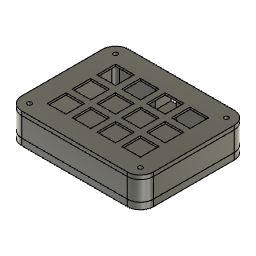
Final_Project (Autodesk Fusion 360 design; units mm, degrees)
Autodesk Fusion 360 part; units mm, degrees
note: some values were not read from the file. Chosen so that the rebuilt part matches the saved one: which bodies a step acts on.
sketch "Sketch1" plane through (0, 0, 0) normal (0, 0, 1) x (1, 0, 0)
  line L0 (-50.425, 81.85) -> (50.425, 81.85)
  line L1 (50.425, 81.85) -> (50.425, 0)
  line L2 (50.425, 0) -> (-50.425, 0)
  line L3 (-50.425, 0) -> (-50.425, 81.85)
  line L4 (-35.425, 28.85) -> (-21.575, 28.85)
  line L5 (-21.575, 28.85) -> (-21.575, 15)
  line L6 (-21.575, 15) -> (-35.425, 15)
  line L7 (-35.425, 15) -> (-35.425, 28.85)
  line L8 (-16.425, 28.85) -> (-2.575, 28.85)
  line L9 (-2.575, 28.85) -> (-2.575, 15)
  line L10 (-2.575, 15) -> (-16.425, 15)
  line L11 (-16.425, 15) -> (-16.425, 28.85)
  line L12 (2.575, 28.85) -> (16.425, 28.85)
  line L13 (16.425, 28.85) -> (16.425, 15)
  line L14 (16.425, 15) -> (2.575, 15)
  line L15 (2.575, 15) -> (2.575, 28.85)
  line L16 (21.575, 28.85) -> (35.425, 28.85)
  line L17 (35.425, 28.85) -> (35.425, 15)
  line L18 (35.425, 15) -> (21.575, 15)
  line L19 (21.575, 15) -> (21.575, 28.85)
  line L20 (-35.425, 47.85) -> (-21.575, 47.85)
  line L21 (-21.575, 47.85) -> (-21.575, 34)
  line L22 (-21.575, 34) -> (-35.425, 34)
  line L23 (-35.425, 34) -> (-35.425, 47.85)
  line L24 (-16.425, 47.85) -> (-2.575, 47.85)
  line L25 (-2.575, 47.85) -> (-2.575, 34)
  line L26 (-2.575, 34) -> (-16.425, 34)
  line L27 (-16.425, 34) -> (-16.425, 47.85)
  line L28 (2.575, 47.85) -> (16.425, 47.85)
  line L29 (16.425, 47.85) -> (16.425, 34)
  line L30 (16.425, 34) -> (2.575, 34)
  line L31 (2.575, 34) -> (2.575, 47.85)
  line L32 (21.575, 47.85) -> (35.425, 47.85)
  line L33 (35.425, 47.85) -> (35.425, 34)
  line L34 (35.425, 34) -> (21.575, 34)
  line L35 (21.575, 34) -> (21.575, 47.85)
  line L36 (-35.425, 66.85) -> (-21.575, 66.85)
  line L37 (-21.575, 66.85) -> (-21.575, 53)
  line L38 (-21.575, 53) -> (-35.425, 53)
  line L39 (-35.425, 53) -> (-35.425, 66.85)
  line L40 (-16.425, 66.85) -> (-2.575, 66.85)
  line L41 (-2.575, 66.85) -> (-2.575, 53)
  line L42 (-2.575, 53) -> (-16.425, 53)
  line L43 (-16.425, 53) -> (-16.425, 66.85)
  line L44 (2.575, 66.85) -> (16.425, 66.85)
  line L45 (16.425, 66.85) -> (16.425, 53)
  line L46 (16.425, 53) -> (2.575, 53)
  line L47 (2.575, 53) -> (2.575, 66.85)
  line L48 (21.575, 66.85) -> (35.425, 66.85)
  line L49 (35.425, 66.85) -> (35.425, 53)
  line L50 (35.425, 53) -> (21.575, 53)
  line L51 (21.575, 53) -> (21.575, 66.85)
  dimension "d1" = 13.85
  dimension "d2" = 13.85
  dimension "d3" = 15
  dimension "d4" = 15
  dimension "d7" = 19
  dimension "d8" = 19
  dimension "d9" = 15
  dimension "d10" = 15
  constraint horizontal L0
  constraint vertical L1
  constraint horizontal L2
  constraint vertical L3
  constraint midpoint origin L2
  constraint horizontal L4
  constraint vertical L5
  constraint horizontal L6
  constraint vertical L7
  measures "d1" distance of L4.start L4.end
  measures "d2" distance of L4.start L6.end
  measures "d3" distance of L2 L6
  measures "d4" distance of L3 L7
  measures "d9" distance of L1 L17
  measures "d10" distance of L0 L48
extrude "Extrude1" add sketch "Sketch1" along normal blind 3 makes body 1
fillet "Fillet1" radius 10 4 edges at (50.425, 0, 1.5) (-50.425, 0, 1.5) (-50.425, 81.85, 1.5) (50.425, 81.85, 1.5) on bodies 1
sketch "Sketch2" plane through (0, 0, 3) normal (0, 0, 1) x (-1, 0, 0)
  arc A0 (-50.425, -71.85) -> (-40.425, -81.85) centre (-40.425, -71.85) ccw
  line L0 (-40.425, -81.85) -> (40.425, -81.85)
  arc A1 (40.425, -81.85) -> (50.425, -71.85) centre (40.425, -71.85) ccw
  line L1 (50.425, -71.85) -> (50.425, -10)
  arc A2 (50.425, -10) -> (40.425, 0) centre (40.425, -10) ccw
  line L2 (40.425, 0) -> (-40.425, 0)
  arc A3 (-40.425, 0) -> (-50.425, -10) centre (-40.425, -10) ccw
  line L3 (-50.425, -10) -> (-50.425, -71.85)
  line L4 (2.575, -34) -> (16.425, -34)
  line L5 (16.425, -34) -> (16.425, -47.85)
  line L6 (16.425, -47.85) -> (2.575, -47.85)
  line L7 (2.575, -47.85) -> (2.575, -34)
  line L8 (-16.425, -15) -> (-2.575, -15)
  line L9 (-2.575, -15) -> (-2.575, -28.85)
  line L10 (-2.575, -28.85) -> (-16.425, -28.85)
  line L11 (-16.425, -28.85) -> (-16.425, -15)
  line L12 (-35.425, -15) -> (-21.575, -15)
  line L13 (-21.575, -15) -> (-21.575, -28.85)
  line L14 (-21.575, -28.85) -> (-35.425, -28.85)
  line L15 (-35.425, -28.85) -> (-35.425, -15)
  line L16 (21.575, -34) -> (35.425, -34)
  line L17 (35.425, -34) -> (35.425, -47.85)
  line L18 (35.425, -47.85) -> (21.575, -47.85)
  line L19 (21.575, -47.85) -> (21.575, -34)
  line L20 (2.575, -15) -> (16.425, -15)
  line L21 (16.425, -15) -> (16.425, -28.85)
  line L22 (16.425, -28.85) -> (2.575, -28.85)
  line L23 (2.575, -28.85) -> (2.575, -15)
  line L24 (21.575, -15) -> (35.425, -15)
  line L25 (35.425, -15) -> (35.425, -28.85)
  line L26 (35.425, -28.85) -> (21.575, -28.85)
  line L27 (21.575, -28.85) -> (21.575, -15)
  line L28 (-16.425, -34) -> (-2.575, -34)
  line L29 (-2.575, -34) -> (-2.575, -47.85)
  line L30 (-2.575, -47.85) -> (-16.425, -47.85)
  line L31 (-16.425, -47.85) -> (-16.425, -34)
  line L32 (-35.425, -34) -> (-21.575, -34)
  line L33 (-21.575, -34) -> (-21.575, -47.85)
  line L34 (-21.575, -47.85) -> (-35.425, -47.85)
  line L35 (-35.425, -47.85) -> (-35.425, -34)
  line L36 (21.575, -53) -> (35.425, -53)
  line L37 (35.425, -53) -> (35.425, -66.85)
  line L38 (35.425, -66.85) -> (21.575, -66.85)
  line L39 (21.575, -66.85) -> (21.575, -53)
  line L40 (2.575, -53) -> (16.425, -53)
  line L41 (16.425, -53) -> (16.425, -66.85)
  line L42 (16.425, -66.85) -> (2.575, -66.85)
  line L43 (2.575, -66.85) -> (2.575, -53)
  line L44 (-16.425, -53) -> (-2.575, -53)
  line L45 (-2.575, -53) -> (-2.575, -66.85)
  line L46 (-2.575, -66.85) -> (-16.425, -66.85)
  line L47 (-16.425, -66.85) -> (-16.425, -53)
  line L48 (-35.425, -53) -> (-21.575, -53)
  line L49 (-21.575, -53) -> (-21.575, -66.85)
  line L50 (-21.575, -66.85) -> (-35.425, -66.85)
  line L51 (-35.425, -66.85) -> (-35.425, -53)
  line L52 (42.425, -73.85) -> (-42.425, -73.85) construction
  line L53 (-42.425, -73.85) -> (-42.425, -8) construction
  line L54 (-42.425, -8) -> (42.425, -8) construction
  line L55 (42.425, -8) -> (42.425, -73.85) construction
  point P0 (42.425, -73.85)
  point P1 (-42.425, -73.85)
  point P2 (-42.425, -8)
  point P3 (42.425, -8)
  dimension "d15" = 8
  dimension "d16" = 8
  dimension "d17" = 8
  dimension "d18" = 8
  constraint horizontal L52
  constraint vertical L53
  constraint horizontal L54
  constraint vertical L55
  constraint coincident P0 L52.start
  constraint coincident P1 L52.end
  constraint coincident P2 L53.end
  constraint coincident P3 L54.end
  measures "d15" distance of L0 L52
  measures "d16" distance of L3 L53
  measures "d17" distance of L2 L54
  measures "d18" distance of L1 L55
hole "Hole1" at (-42.425, 73.85, 3) at (-42.425, 8, 3) at (42.425, 8, 3) at (42.425, 73.85, 3) direction (0, 0, -1) diameter 3.2 depth 20 tip angle 118 bodies 1
sketch "Sketch3" plane through (0, 0, 3) normal (0, 0, 1) x (-1, 0, 0)
  circle A0 centre (-42.425, -8) radius 1.6
  circle A1 centre (42.425, -73.85) radius 1.6
  circle A2 centre (42.425, -8) radius 1.6
  circle A3 centre (-42.425, -73.85) radius 1.6
  arc A4 (-50.425, -71.85) -> (-40.425, -81.85) centre (-40.425, -71.85) ccw
  line L0 (-40.425, -81.85) -> (40.425, -81.85)
  arc A5 (40.425, -81.85) -> (50.425, -71.85) centre (40.425, -71.85) ccw
  line L1 (50.425, -71.85) -> (50.425, -10)
  arc A6 (50.425, -10) -> (40.425, 0) centre (40.425, -10) ccw
  line L2 (40.425, 0) -> (-40.425, 0)
  arc A7 (-40.425, 0) -> (-50.425, -10) centre (-40.425, -10) ccw
  line L3 (-50.425, -10) -> (-50.425, -71.85)
  line L4 (-16.425, -53) -> (-2.575, -53)
  line L5 (-2.575, -53) -> (-2.575, -66.85)
  line L6 (-2.575, -66.85) -> (-16.425, -66.85)
  line L7 (-16.425, -66.85) -> (-16.425, -53)
  line L8 (2.575, -53) -> (16.425, -53)
  line L9 (16.425, -53) -> (16.425, -66.85)
  line L10 (16.425, -66.85) -> (2.575, -66.85)
  line L11 (2.575, -66.85) -> (2.575, -53)
  line L12 (21.575, -53) -> (35.425, -53)
  line L13 (35.425, -53) -> (35.425, -66.85)
  line L14 (35.425, -66.85) -> (21.575, -66.85)
  line L15 (21.575, -66.85) -> (21.575, -53)
  line L16 (-35.425, -34) -> (-21.575, -34)
  line L17 (-21.575, -34) -> (-21.575, -47.85)
  line L18 (-21.575, -47.85) -> (-35.425, -47.85)
  line L19 (-35.425, -47.85) -> (-35.425, -34)
  line L20 (-35.425, -53) -> (-21.575, -53)
  line L21 (-21.575, -53) -> (-21.575, -66.85)
  line L22 (-21.575, -66.85) -> (-35.425, -66.85)
  line L23 (-35.425, -66.85) -> (-35.425, -53)
  line L24 (21.575, -34) -> (35.425, -34)
  line L25 (35.425, -34) -> (35.425, -47.85)
  line L26 (35.425, -47.85) -> (21.575, -47.85)
  line L27 (21.575, -47.85) -> (21.575, -34)
  line L28 (-16.425, -34) -> (-2.575, -34)
  line L29 (-2.575, -34) -> (-2.575, -47.85)
  line L30 (-2.575, -47.85) -> (-16.425, -47.85)
  line L31 (-16.425, -47.85) -> (-16.425, -34)
  line L32 (2.575, -34) -> (16.425, -34)
  line L33 (16.425, -34) -> (16.425, -47.85)
  line L34 (16.425, -47.85) -> (2.575, -47.85)
  line L35 (2.575, -47.85) -> (2.575, -34)
  line L36 (-35.425, -15) -> (-21.575, -15)
  line L37 (-21.575, -15) -> (-21.575, -28.85)
  line L38 (-21.575, -28.85) -> (-35.425, -28.85)
  line L39 (-35.425, -28.85) -> (-35.425, -15)
  line L40 (-16.425, -15) -> (-2.575, -15)
  line L41 (-2.575, -15) -> (-2.575, -28.85)
  line L42 (-2.575, -28.85) -> (-16.425, -28.85)
  line L43 (-16.425, -28.85) -> (-16.425, -15)
  line L44 (2.575, -15) -> (16.425, -15)
  line L45 (16.425, -15) -> (16.425, -28.85)
  line L46 (16.425, -28.85) -> (2.575, -28.85)
  line L47 (2.575, -28.85) -> (2.575, -15)
  line L48 (21.575, -15) -> (35.425, -15)
  line L49 (35.425, -15) -> (35.425, -28.85)
  line L50 (35.425, -28.85) -> (21.575, -28.85)
  line L51 (21.575, -28.85) -> (21.575, -15)
sketch "Sketch4" plane through (0, 0, 0) normal (0, 0, -1) x (1, 0, 0)
  circle A0 centre (42.425, -8) radius 1.6
  circle A1 centre (-42.425, -73.85) radius 1.6
  circle A2 centre (-42.425, -8) radius 1.6
  circle A3 centre (42.425, -73.85) radius 1.6
  line L0 (2.575, -53) -> (16.425, -53)
  line L1 (16.425, -53) -> (16.425, -66.85)
  line L2 (16.425, -66.85) -> (2.575, -66.85)
  line L3 (2.575, -66.85) -> (2.575, -53)
  line L4 (21.575, -53) -> (35.425, -53)
  line L5 (35.425, -53) -> (35.425, -66.85)
  line L6 (35.425, -66.85) -> (21.575, -66.85)
  line L7 (21.575, -66.85) -> (21.575, -53)
  line L8 (-16.425, -53) -> (-2.575, -53)
  line L9 (-2.575, -53) -> (-2.575, -66.85)
  line L10 (-2.575, -66.85) -> (-16.425, -66.85)
  line L11 (-16.425, -66.85) -> (-16.425, -53)
  line L12 (-35.425, -53) -> (-21.575, -53)
  line L13 (-21.575, -53) -> (-21.575, -66.85)
  line L14 (-21.575, -66.85) -> (-35.425, -66.85)
  line L15 (-35.425, -66.85) -> (-35.425, -53)
  line L16 (21.575, -34) -> (35.425, -34)
  line L17 (35.425, -34) -> (35.425, -47.85)
  line L18 (35.425, -47.85) -> (21.575, -47.85)
  line L19 (21.575, -47.85) -> (21.575, -34)
  line L20 (2.575, -34) -> (16.425, -34)
  line L21 (16.425, -34) -> (16.425, -47.85)
  line L22 (16.425, -47.85) -> (2.575, -47.85)
  line L23 (2.575, -47.85) -> (2.575, -34)
  line L24 (-16.425, -34) -> (-2.575, -34)
  line L25 (-2.575, -34) -> (-2.575, -47.85)
  line L26 (-2.575, -47.85) -> (-16.425, -47.85)
  line L27 (-16.425, -47.85) -> (-16.425, -34)
  line L28 (-35.425, -15) -> (-21.575, -15)
  line L29 (-21.575, -15) -> (-21.575, -28.85)
  line L30 (-21.575, -28.85) -> (-35.425, -28.85)
  line L31 (-35.425, -28.85) -> (-35.425, -15)
  line L32 (-35.425, -34) -> (-21.575, -34)
  line L33 (-21.575, -34) -> (-21.575, -47.85)
  line L34 (-21.575, -47.85) -> (-35.425, -47.85)
  line L35 (-35.425, -47.85) -> (-35.425, -34)
  line L36 (21.575, -15) -> (35.425, -15)
  line L37 (35.425, -15) -> (35.425, -28.85)
  line L38 (35.425, -28.85) -> (21.575, -28.85)
  line L39 (21.575, -28.85) -> (21.575, -15)
  line L40 (-16.425, -15) -> (-2.575, -15)
  line L41 (-2.575, -15) -> (-2.575, -28.85)
  line L42 (-2.575, -28.85) -> (-16.425, -28.85)
  line L43 (-16.425, -28.85) -> (-16.425, -15)
  line L44 (2.575, -15) -> (16.425, -15)
  line L45 (16.425, -15) -> (16.425, -28.85)
  line L46 (16.425, -28.85) -> (2.575, -28.85)
  line L47 (2.575, -28.85) -> (2.575, -15)
  arc A4 (40.425, -81.85) -> (50.425, -71.85) centre (42.425, -73.85) ccw
  line L48 (50.425, -71.85) -> (50.425, -10)
  arc A5 (50.425, -10) -> (40.425, 0) centre (42.425, -8) ccw
  line L49 (40.425, 0) -> (-40.425, 0)
  arc A6 (-40.425, 0) -> (-50.425, -10) centre (-42.425, -8) ccw
  line L50 (-50.425, -10) -> (-50.425, -71.85)
  arc A7 (-50.425, -71.85) -> (-40.425, -81.85) centre (-42.425, -73.85) ccw
  line L51 (-40.425, -81.85) -> (40.425, -81.85)
  point P0 (40.425, -71.85)
  point P1 (40.425, -10)
  point P2 (-40.425, -10)
  point P3 (-40.425, -71.85)
  point P4 (40.425, -71.85)
  point P5 (40.425, -10)
  point P6 (-40.425, -10)
  point P7 (-40.425, -71.85)
  point P8 (40.425, -71.85)
  point P9 (40.425, -10)
  point P10 (-40.425, -10)
  point P11 (-40.425, -71.85)
extrude "Extrude2" add sketch "Sketch4" along normal blind 20 separate body contours A0 | A1 | A2 | A3 | L0 L1 L2 L3 | L4 L5 L6 L7 | L8 L9 L10 L11 | L12 L13 L14 L15 | L16 L17 L18 L19 | L20 L21 L22 L23 | L24 L25 L26 L27 | L28 L29 L30 L31 | L32 L33 L34 L35 | L36 L37 L38 L39 | L40 L41 L42 L43 | L44 L45 L46 L47 | A4 L48 A5 L49 A6 L50 A7 L51 makes body 2
sketch "Sketch5" plane through (0, 0, 0) normal (0, 0, 1) x (-1, 0, 0)
  line L0 (-40.425, -81.85) -> (40.425, -81.85)
  arc A0 (40.425, -81.85) -> (50.425, -71.85) centre (42.425, -73.85) ccw
  line L1 (50.425, -71.85) -> (50.425, -10)
  arc A1 (50.425, -10) -> (40.425, 0) centre (42.425, -8) ccw
  line L2 (40.425, 0) -> (-40.425, 0)
  arc A2 (-40.425, 0) -> (-50.425, -10) centre (-42.425, -8) ccw
  line L3 (-50.425, -10) -> (-50.425, -71.85)
  arc A3 (-50.425, -71.85) -> (-40.425, -81.85) centre (-42.425, -73.85) ccw
  line L4 (38.425, -69.85) -> (-38.425, -69.85)
  line L5 (-38.425, -69.85) -> (-38.425, -12)
  line L6 (-38.425, -12) -> (38.425, -12)
  line L7 (38.425, -12) -> (38.425, -69.85)
  dimension "d24" = 12
  dimension "d25" = 12
  dimension "d26" = 12
  dimension "d27" = 12
  constraint horizontal L4
  constraint vertical L5
  constraint horizontal L6
  constraint vertical L7
  measures "d24" distance of L0 L4
  measures "d25" distance of L3 L5
  measures "d26" distance of L2 L6
  measures "d27" distance of L1 L7
extrude "Extrude3" cut sketch "Sketch5" against normal blind 15 contours L4 L5 L6 L7 bodies 2
fillet "Fillet2" radius 3 4 edges at (-38.425, 69.85, -7.5) (38.425, 69.85, -7.5) (38.425, 12, -7.5) (-38.425, 12, -7.5) on bodies 2
sketch "Sketch6" plane through (0, 0, 0) normal (0, 0, 1) x (-1, 0, 0)
  line L0 (-38.425, -66.85) -> (-38.425, -15)
  arc A0 (-35.425, -12) -> (-38.425, -15) centre (-35.425, -15) ccw
  line L1 (-35.425, -12) -> (35.425, -12)
  arc A1 (38.425, -15) -> (35.425, -12) centre (35.425, -15) ccw
  line L2 (38.425, -15) -> (38.425, -66.85)
  arc A2 (35.425, -69.85) -> (38.425, -66.85) centre (35.425, -66.85) ccw
  line L3 (35.425, -69.85) -> (-35.425, -69.85)
  arc A3 (-38.425, -66.85) -> (-35.425, -69.85) centre (-35.425, -66.85) ccw
  line L4 (-40.425, -81.85) -> (40.425, -81.85)
  arc A4 (40.425, -81.85) -> (50.425, -71.85) centre (42.425, -73.85) ccw
  line L5 (50.425, -71.85) -> (50.425, -10)
  arc A5 (50.425, -10) -> (40.425, 0) centre (42.425, -8) ccw
  line L6 (40.425, 0) -> (-40.425, 0)
  arc A6 (-40.425, 0) -> (-50.425, -10) centre (-42.425, -8) ccw
  line L7 (-50.425, -10) -> (-50.425, -71.85)
  arc A7 (-50.425, -71.85) -> (-40.425, -81.85) centre (-42.425, -73.85) ccw
  point P0 (42.425, -73.85)
  point P1 (-42.425, -73.85)
  point P2 (-42.425, -8)
  point P3 (42.425, -8)
  constraint coincident P0 A4.centre
  constraint coincident P1 A7.centre
  constraint coincident P2 A6.centre
  constraint coincident P3 A5.centre
sketch "Sketch7" plane through (0, 0, 0) normal (0, 0, 1) x (-1, 0, 0)
  line L0 (-38.425, -66.85) -> (-38.425, -15)
  arc A0 (-35.425, -12) -> (-38.425, -15) centre (-35.425, -15) ccw
  line L1 (-35.425, -12) -> (35.425, -12)
  arc A1 (38.425, -15) -> (35.425, -12) centre (35.425, -15) ccw
  line L2 (38.425, -15) -> (38.425, -66.85)
  arc A2 (35.425, -69.85) -> (38.425, -66.85) centre (35.425, -66.85) ccw
  line L3 (35.425, -69.85) -> (-35.425, -69.85)
  arc A3 (-38.425, -66.85) -> (-35.425, -69.85) centre (-35.425, -66.85) ccw
  line L4 (-40.425, -81.85) -> (40.425, -81.85)
  arc A4 (40.425, -81.85) -> (50.425, -71.85) centre (42.425, -73.85) ccw
  line L5 (50.425, -71.85) -> (50.425, -10)
  arc A5 (50.425, -10) -> (40.425, 0) centre (42.425, -8) ccw
  line L6 (40.425, 0) -> (-40.425, 0)
  arc A6 (-40.425, 0) -> (-50.425, -10) centre (-42.425, -8) ccw
  line L7 (-50.425, -10) -> (-50.425, -71.85)
  arc A7 (-50.425, -71.85) -> (-40.425, -81.85) centre (-42.425, -73.85) ccw
  line L8 (8, -81.85) -> (-8, -81.85)
  line L9 (-8, -81.85) -> (-8, -69.85)
  line L10 (-8, -69.85) -> (8, -69.85)
  line L11 (8, -69.85) -> (8, -81.85)
  dimension "d35" = 16
  constraint horizontal L8
  constraint vertical L9
  constraint horizontal L10
  constraint vertical L11
  constraint coincident L3 L9.end
  constraint coincident L4 L8.start
  constraint midpoint L4 L8
  measures "d35" distance of L8.start L8.end
extrude "Extrude4" cut sketch "Sketch7" against normal blind 15 contours L0 A0 L1 A1 L2 A2 L3 A3 L10 | L3 L4 L8 L9 L10 L11 bodies 2
extrude "Extrude5" cut 1 faces at (13.475, 54.5667, -20) along direction (0, 0, 1) blind 2 on bodies 2 bodies 2
sketch "Sketch8" plane through (0, 0, -15) normal (0, 0, 1) x (-1, 0, 0)
  arc A0 (38.425, -15) -> (35.425, -12) centre (35.425, -15) ccw
  line L0 (35.425, -12) -> (-35.425, -12)
  arc A1 (-35.425, -12) -> (-38.425, -15) centre (-35.425, -15) ccw
  line L1 (-38.425, -15) -> (-38.425, -66.85)
  arc A2 (-38.425, -66.85) -> (-35.425, -69.85) centre (-35.425, -66.85) ccw
  line L2 (-35.425, -69.85) -> (-8, -69.85)
  line L3 (-8, -69.85) -> (-8, -81.85)
  line L4 (-8, -81.85) -> (8, -81.85)
  line L5 (8, -81.85) -> (8, -69.85)
  line L6 (8, -69.85) -> (35.425, -69.85)
  arc A3 (35.425, -69.85) -> (38.425, -66.85) centre (35.425, -66.85) ccw
  line L7 (38.425, -66.85) -> (38.425, -15)
sketch "Sketch9" plane through (0, 0, -18) normal (0, 0, -1) x (1, 0, 0)
  line L0 (-40.425, -81.85) -> (40.425, -81.85)
  arc A0 (40.425, -81.85) -> (50.425, -71.85) centre (42.425, -73.85) ccw
  line L1 (50.425, -71.85) -> (50.425, -10)
  arc A1 (50.425, -10) -> (40.425, 0) centre (42.425, -8) ccw
  line L2 (40.425, 0) -> (-40.425, 0)
  arc A2 (-40.425, 0) -> (-50.425, -10) centre (-42.425, -8) ccw
  line L3 (-50.425, -10) -> (-50.425, -71.85)
  arc A3 (-50.425, -71.85) -> (-40.425, -81.85) centre (-42.425, -73.85) ccw
sketch "Sketch10" plane through (0, 0, 0) normal (0, 0, 1) x (-1, 0, 0)
  line L0 (-8, -81.85) -> (-8, -69.85)
  line L1 (-8, -69.85) -> (-35.425, -69.85)
  arc A0 (-38.425, -66.85) -> (-35.425, -69.85) centre (-35.425, -66.85) ccw
  line L2 (-38.425, -66.85) -> (-38.425, -15)
  arc A1 (-35.425, -12) -> (-38.425, -15) centre (-35.425, -15) ccw
  line L3 (-35.425, -12) -> (35.425, -12)
  arc A2 (38.425, -15) -> (35.425, -12) centre (35.425, -15) ccw
  line L4 (38.425, -15) -> (38.425, -66.85)
  arc A3 (35.425, -69.85) -> (38.425, -66.85) centre (35.425, -66.85) ccw
  line L5 (35.425, -69.85) -> (8, -69.85)
  line L6 (8, -69.85) -> (8, -81.85)
  line L7 (8, -81.85) -> (40.425, -81.85)
  arc A4 (40.425, -81.85) -> (50.425, -71.85) centre (42.425, -73.85) ccw
  line L8 (50.425, -71.85) -> (50.425, -10)
  arc A5 (50.425, -10) -> (40.425, 0) centre (42.425, -8) ccw
  line L9 (40.425, 0) -> (-40.425, 0)
  arc A6 (-40.425, 0) -> (-50.425, -10) centre (-42.425, -8) ccw
  line L10 (-50.425, -10) -> (-50.425, -71.85)
  arc A7 (-50.425, -71.85) -> (-40.425, -81.85) centre (-42.425, -73.85) ccw
  line L11 (-40.425, -81.85) -> (-8, -81.85)
sketch "Sketch11" plane through (0, 0, 0) normal (0, 0, -1) x (1, 0, 0)
  circle A0 centre (42.425, -8) radius 1.6
  circle A1 centre (-42.425, -73.85) radius 1.6
  circle A2 centre (-42.425, -8) radius 1.6
  circle A3 centre (42.425, -73.85) radius 1.6
  line L0 (-35.425, -15) -> (-21.575, -15)
  line L1 (-21.575, -15) -> (-21.575, -28.85)
  line L2 (-21.575, -28.85) -> (-35.425, -28.85)
  line L3 (-35.425, -28.85) -> (-35.425, -15)
  line L4 (-16.425, -53) -> (-2.575, -53)
  line L5 (-2.575, -53) -> (-2.575, -66.85)
  line L6 (-2.575, -66.85) -> (-16.425, -66.85)
  line L7 (-16.425, -66.85) -> (-16.425, -53)
  line L8 (2.575, -53) -> (16.425, -53)
  line L9 (16.425, -53) -> (16.425, -66.85)
  line L10 (16.425, -66.85) -> (2.575, -66.85)
  line L11 (2.575, -66.85) -> (2.575, -53)
  line L12 (21.575, -53) -> (35.425, -53)
  line L13 (35.425, -53) -> (35.425, -66.85)
  line L14 (35.425, -66.85) -> (21.575, -66.85)
  line L15 (21.575, -66.85) -> (21.575, -53)
  line L16 (-35.425, -53) -> (-21.575, -53)
  line L17 (-21.575, -53) -> (-21.575, -66.85)
  line L18 (-21.575, -66.85) -> (-35.425, -66.85)
  line L19 (-35.425, -66.85) -> (-35.425, -53)
  line L20 (21.575, -34) -> (35.425, -34)
  line L21 (35.425, -34) -> (35.425, -47.85)
  line L22 (35.425, -47.85) -> (21.575, -47.85)
  line L23 (21.575, -47.85) -> (21.575, -34)
  line L24 (2.575, -34) -> (16.425, -34)
  line L25 (16.425, -34) -> (16.425, -47.85)
  line L26 (16.425, -47.85) -> (2.575, -47.85)
  line L27 (2.575, -47.85) -> (2.575, -34)
  line L28 (-16.425, -34) -> (-2.575, -34)
  line L29 (-2.575, -34) -> (-2.575, -47.85)
  line L30 (-2.575, -47.85) -> (-16.425, -47.85)
  line L31 (-16.425, -47.85) -> (-16.425, -34)
  line L32 (-35.425, -34) -> (-21.575, -34)
  line L33 (-21.575, -34) -> (-21.575, -47.85)
  line L34 (-21.575, -47.85) -> (-35.425, -47.85)
  line L35 (-35.425, -47.85) -> (-35.425, -34)
  line L36 (21.575, -15) -> (35.425, -15)
  line L37 (35.425, -15) -> (35.425, -28.85)
  line L38 (35.425, -28.85) -> (21.575, -28.85)
  line L39 (21.575, -28.85) -> (21.575, -15)
  line L40 (2.575, -15) -> (16.425, -15)
  line L41 (16.425, -15) -> (16.425, -28.85)
  line L42 (16.425, -28.85) -> (2.575, -28.85)
  line L43 (2.575, -28.85) -> (2.575, -15)
  line L44 (-16.425, -15) -> (-2.575, -15)
  line L45 (-2.575, -15) -> (-2.575, -28.85)
  line L46 (-2.575, -28.85) -> (-16.425, -28.85)
  line L47 (-16.425, -28.85) -> (-16.425, -15)
  arc A4 (40.425, -81.85) -> (50.425, -71.85) centre (42.425, -73.85) ccw
  line L48 (50.425, -71.85) -> (50.425, -10)
  arc A5 (50.425, -10) -> (40.425, 0) centre (42.425, -8) ccw
  line L49 (40.425, 0) -> (-40.425, 0)
  arc A6 (-40.425, 0) -> (-50.425, -10) centre (-42.425, -8) ccw
  line L50 (-50.425, -10) -> (-50.425, -71.85)
  arc A7 (-50.425, -71.85) -> (-40.425, -81.85) centre (-42.425, -73.85) ccw
  line L51 (-40.425, -81.85) -> (40.425, -81.85)
  line L52 (-37.425, -13) -> (37.425, -13)
  line L53 (37.425, -13) -> (37.425, -68.85)
  line L54 (37.425, -68.85) -> (-37.425, -68.85)
  line L55 (-37.425, -68.85) -> (-37.425, -13)
  point P0 (40.425, -71.85)
  point P1 (40.425, -10)
  point P2 (-40.425, -10)
  point P3 (-40.425, -71.85)
  point P4 (40.425, -71.85)
  point P5 (40.425, -10)
  point P6 (-40.425, -10)
  point P7 (-40.425, -71.85)
  point P8 (40.425, -71.85)
  point P9 (40.425, -10)
  point P10 (-40.425, -10)
  point P11 (-40.425, -71.85)
  dimension "d40" = 2
  dimension "d41" = 2
  dimension "d42" = 2
  dimension "d43" = 2
  constraint horizontal L52
  constraint vertical L53
  constraint horizontal L54
  constraint vertical L55
  measures "d40" distance of L0 L52
  measures "d41" distance of L3 L55
  measures "d42" distance of L18 L54
  measures "d43" distance of L13 L53
extrude "Extrude6" cut sketch "Sketch11" against normal blind 1.5 contours L52 L53 L54 L55 bodies 1
sketch "Sketch12" plane through (0, 0, 3) normal (0, 0, 1) x (-1, 0, 0)
  circle A0 centre (-42.425, -8) radius 1.6
  circle A1 centre (42.425, -73.85) radius 1.6
  circle A2 centre (42.425, -8) radius 1.6
  circle A3 centre (-42.425, -73.85) radius 1.6
  arc A4 (-50.425, -71.85) -> (-40.425, -81.85) centre (-42.425, -73.85) ccw
  line L0 (-40.425, -81.85) -> (40.425, -81.85)
  arc A5 (40.425, -81.85) -> (50.425, -71.85) centre (42.425, -73.85) ccw
  line L1 (50.425, -71.85) -> (50.425, -10)
  arc A6 (50.425, -10) -> (40.425, 0) centre (42.425, -8) ccw
  line L2 (40.425, 0) -> (-40.425, 0)
  arc A7 (-40.425, 0) -> (-50.425, -10) centre (-42.425, -8) ccw
  line L3 (-50.425, -10) -> (-50.425, -71.85)
  line L4 (21.575, -15) -> (35.425, -15)
  line L5 (35.425, -15) -> (35.425, -28.85)
  line L6 (35.425, -28.85) -> (21.575, -28.85)
  line L7 (21.575, -28.85) -> (21.575, -15)
  line L8 (2.575, -53) -> (16.425, -53)
  line L9 (16.425, -53) -> (16.425, -66.85)
  line L10 (16.425, -66.85) -> (2.575, -66.85)
  line L11 (2.575, -66.85) -> (2.575, -53)
  line L12 (-16.425, -53) -> (-2.575, -53)
  line L13 (-2.575, -53) -> (-2.575, -66.85)
  line L14 (-2.575, -66.85) -> (-16.425, -66.85)
  line L15 (-16.425, -66.85) -> (-16.425, -53)
  line L16 (-35.425, -53) -> (-21.575, -53)
  line L17 (-21.575, -53) -> (-21.575, -66.85)
  line L18 (-21.575, -66.85) -> (-35.425, -66.85)
  line L19 (-35.425, -66.85) -> (-35.425, -53)
  line L20 (21.575, -53) -> (35.425, -53)
  line L21 (35.425, -53) -> (35.425, -66.85)
  line L22 (35.425, -66.85) -> (21.575, -66.85)
  line L23 (21.575, -66.85) -> (21.575, -53)
  line L24 (-35.425, -34) -> (-21.575, -34)
  line L25 (-21.575, -34) -> (-21.575, -47.85)
  line L26 (-21.575, -47.85) -> (-35.425, -47.85)
  line L27 (-35.425, -47.85) -> (-35.425, -34)
  line L28 (-16.425, -34) -> (-2.575, -34)
  line L29 (-2.575, -34) -> (-2.575, -47.85)
  line L30 (-2.575, -47.85) -> (-16.425, -47.85)
  line L31 (-16.425, -47.85) -> (-16.425, -34)
  line L32 (2.575, -34) -> (16.425, -34)
  line L33 (16.425, -34) -> (16.425, -47.85)
  line L34 (16.425, -47.85) -> (2.575, -47.85)
  line L35 (2.575, -47.85) -> (2.575, -34)
  line L36 (21.575, -34) -> (35.425, -34)
  line L37 (35.425, -34) -> (35.425, -47.85)
  line L38 (35.425, -47.85) -> (21.575, -47.85)
  line L39 (21.575, -47.85) -> (21.575, -34)
  line L40 (-35.425, -15) -> (-21.575, -15)
  line L41 (-21.575, -15) -> (-21.575, -28.85)
  line L42 (-21.575, -28.85) -> (-35.425, -28.85)
  line L43 (-35.425, -28.85) -> (-35.425, -15)
  line L44 (-16.425, -15) -> (-2.575, -15)
  line L45 (-2.575, -15) -> (-2.575, -28.85)
  line L46 (-2.575, -28.85) -> (-16.425, -28.85)
  line L47 (-16.425, -28.85) -> (-16.425, -15)
  line L48 (2.575, -15) -> (16.425, -15)
  line L49 (16.425, -15) -> (16.425, -28.85)
  line L50 (16.425, -28.85) -> (2.575, -28.85)
  line L51 (2.575, -28.85) -> (2.575, -15)
  line L52 (35.6, -67.025) -> (21.4, -67.025)
  line L53 (21.4, -67.025) -> (21.4, -52.825)
  line L54 (21.4, -52.825) -> (35.6, -52.825)
  line L55 (35.6, -52.825) -> (35.6, -67.025)
  line L56 (35.6, -67.025) -> (21.4, -52.825)
  line L57 (35.425, -53) -> (21.575, -66.85)
  point P0 (-40.425, -71.85)
  point P1 (40.425, -71.85)
  point P2 (40.425, -10)
  point P3 (-40.425, -10)
  point P4 (-40.425, -71.85)
  point P5 (40.425, -71.85)
  point P6 (40.425, -10)
  point P7 (-40.425, -10)
  point P8 (-40.425, -71.85)
  point P9 (40.425, -71.85)
  point P10 (40.425, -10)
  point P11 (-40.425, -10)
  dimension "d46" = 14.2
  constraint horizontal L52
  constraint vertical L53
  constraint horizontal L54
  constraint vertical L55
  constraint coincident L20.end L21.start
  constraint coincident L22.end L23.start
  constraint midpoint L56 L57
  constraint equal L52 L55
  measures "d46" distance of L52.start L52.end
extrude "Extrude7" cut sketch "Sketch12" against normal blind 3 contours L20 L21 L54 L55 L56 | L23 L56 L57 | L22 L23 L52 L53 L56 | L20 L56 L57 | L21 L56 L57 | L22 L56 L57 bodies 1
pattern_linear "R-Pattern1" count 4 spacing 19 along (1, 0, 0) count 3 spacing 19 along (0, -1, 0) of "Extrude7"
sketch "Sketch13" plane through (0, 0, 3) normal (0, 0, 1) x (-1, 0, 0)
  line L0 (-35.6, -29.025) -> (-35.6, -14.825)
  line L1 (-35.6, -14.825) -> (-21.4, -14.825)
  line L2 (-21.4, -14.825) -> (-21.4, -29.025)
  line L3 (-21.4, -29.025) -> (-35.6, -29.025)
  line L4 (-16.6, -29.025) -> (-16.6, -14.825)
  line L5 (-16.6, -14.825) -> (-2.4, -14.825)
  line L6 (-2.4, -14.825) -> (-2.4, -29.025)
  line L7 (-2.4, -29.025) -> (-16.6, -29.025)
  line L8 (2.4, -29.025) -> (2.4, -14.825)
  line L9 (2.4, -14.825) -> (16.6, -14.825)
  line L10 (16.6, -14.825) -> (16.6, -29.025)
  line L11 (16.6, -29.025) -> (2.4, -29.025)
  line L12 (21.4, -29.025) -> (21.4, -14.825)
  line L13 (21.4, -14.825) -> (35.6, -14.825)
  line L14 (35.6, -14.825) -> (35.6, -29.025)
  line L15 (35.6, -29.025) -> (21.4, -29.025)
  line L16 (-35.6, -48.025) -> (-35.6, -33.825)
  line L17 (-35.6, -33.825) -> (-21.4, -33.825)
  line L18 (-21.4, -33.825) -> (-21.4, -48.025)
  line L19 (-21.4, -48.025) -> (-35.6, -48.025)
  line L20 (-16.6, -48.025) -> (-16.6, -33.825)
  line L21 (-16.6, -33.825) -> (-2.4, -33.825)
  line L22 (-2.4, -33.825) -> (-2.4, -48.025)
  line L23 (-2.4, -48.025) -> (-16.6, -48.025)
  line L24 (2.4, -48.025) -> (2.4, -33.825)
  line L25 (2.4, -33.825) -> (16.6, -33.825)
  line L26 (16.6, -33.825) -> (16.6, -48.025)
  line L27 (16.6, -48.025) -> (2.4, -48.025)
  line L28 (21.4, -48.025) -> (21.4, -33.825)
  line L29 (21.4, -33.825) -> (35.6, -33.825)
  line L30 (35.6, -33.825) -> (35.6, -48.025)
  line L31 (35.6, -48.025) -> (21.4, -48.025)
  line L32 (-35.6, -67.025) -> (-35.6, -52.825)
  line L33 (-35.6, -52.825) -> (-21.4, -52.825)
  line L34 (-21.4, -52.825) -> (-21.4, -67.025)
  line L35 (-21.4, -67.025) -> (-35.6, -67.025)
  line L36 (-16.6, -67.025) -> (-16.6, -52.825)
  line L37 (-16.6, -52.825) -> (-2.4, -52.825)
  line L38 (-2.4, -52.825) -> (-2.4, -67.025)
  line L39 (-2.4, -67.025) -> (-16.6, -67.025)
  line L40 (2.4, -67.025) -> (2.4, -52.825)
  line L41 (2.4, -52.825) -> (16.6, -52.825)
  line L42 (16.6, -52.825) -> (16.6, -67.025)
  line L43 (16.6, -67.025) -> (2.4, -67.025)
  line L44 (21.4, -67.025) -> (21.4, -52.825)
  line L45 (21.4, -52.825) -> (35.6, -52.825)
  line L46 (35.6, -52.825) -> (35.6, -67.025)
  line L47 (35.6, -67.025) -> (21.4, -67.025)
  circle A0 centre (-42.425, -8) radius 1.6
  circle A1 centre (42.425, -73.85) radius 1.6
  circle A2 centre (42.425, -8) radius 1.6
  circle A3 centre (-42.425, -73.85) radius 1.6
  arc A4 (-50.425, -71.85) -> (-40.425, -81.85) centre (-40.425, -71.85) ccw
  line L48 (-40.425, -81.85) -> (40.425, -81.85)
  arc A5 (40.425, -81.85) -> (50.425, -71.85) centre (40.425, -71.85) ccw
  line L49 (50.425, -71.85) -> (50.425, -10)
  arc A6 (50.425, -10) -> (40.425, 0) centre (40.425, -10) ccw
  line L50 (40.425, 0) -> (-40.425, 0)
  arc A7 (-40.425, 0) -> (-50.425, -10) centre (-40.425, -10) ccw
  line L51 (-50.425, -10) -> (-50.425, -71.85)
  arc A8 (40.425, -81.85) -> (50.425, -71.85) centre (42.425, -73.85) ccw
  arc A9 (-50.425, -71.85) -> (-40.425, -81.85) centre (-42.425, -73.85) ccw
  arc A10 (-40.425, 0) -> (-50.425, -10) centre (-42.425, -8) ccw
  arc A11 (50.425, -10) -> (40.425, 0) centre (42.425, -8) ccw
extrude "Extrude8" cut sketch "Sketch13" against normal blind 21 contours A4 A9 | A7 A10 | A5 A8 | A6 A11 bodies 2
split "Split1" by plane through (0, 0, -15) normal (0, 0, 1) bodies 2 makes body 3 at (11.8083, 4, 0)
extrude "Extrude9" add 1 faces at (13.475, 54.5667, -18) along direction (0, 0, -1) blind 2 on bodies 2 bodies 2
